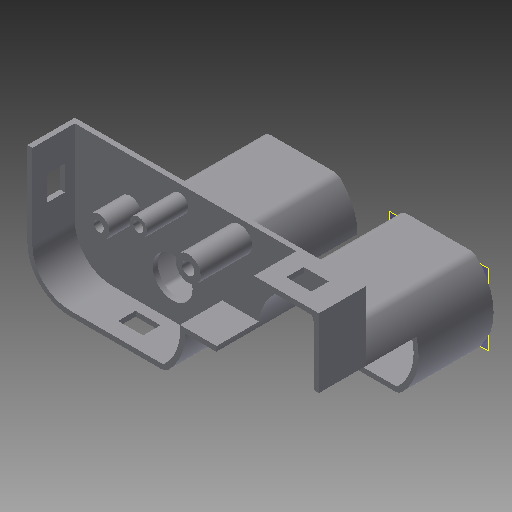
# Autodesk Inventor part: frame1
Saved by Autodesk Inventor 2017 (Build 210142000, 142)
## iProperties
Created: 2017-01-16
Part Number: frame1
Material: Generic
Document SubType Name: Modeling
Designer: Paulo Loma
Density: 1 g/cm^3
Appearance: Default
Author: Paulo Loma
Autodesk Inventor part; units mm, degrees
sketch "Sketch1" plane through (0, 0, 0) normal (0, 0, 1) x (1, 0, 0)
  arc A0 (6.9166, 7.2222) -> (6.2249, 7.5) centre (6.2249, 6.5) ccw projected
  arc A1 (6.9166, -7.2222) -> (6.9166, 7.2222) centre (0, 0) ccw
  arc A2 (6.2249, -7.5) -> (6.9166, -7.2222) centre (6.2249, -6.5) ccw projected
  line L0 (6.2249, -7.5) -> (-6.2249, -7.5)
  arc A3 (-6.9166, -7.2222) -> (-6.2249, -7.5) centre (-6.2249, -6.5) ccw projected
  arc A4 (-6.9166, 7.2222) -> (-6.9166, -7.2222) centre (0, 0) ccw
  arc A5 (-6.2249, 7.5) -> (-6.9166, 7.2222) centre (-6.2249, 6.5) ccw projected
  line L1 (-6.2249, 7.5) -> (6.2249, 7.5)
  arc A6 (-7.6083, -7.9444) -> (-6.2249, -8.5) centre (-6.2249, -6.5) ccw
  line L2 (-6.2249, -8.5) -> (6.2249, -8.5)
  arc A7 (6.2249, -8.5) -> (7.6083, -7.9444) centre (6.2249, -6.5) ccw
  arc A8 (7.6083, -7.9444) -> (7.6083, 7.9444) centre (0, 0) ccw
  arc A9 (7.6083, 7.9444) -> (6.2249, 8.5) centre (6.2249, 6.5) ccw
  line L3 (6.2249, 8.5) -> (-6.2249, 8.5)
  arc A10 (-6.2249, 8.5) -> (-7.6083, 7.9444) centre (-6.2249, 6.5) ccw
  arc A11 (-7.6083, 7.9444) -> (-7.6083, -7.9444) centre (0, 0) ccw
  dimension "d0" = 1
  constraints: 16 point on circle, 8 centre point, 8 end point, 7 other
  measures "d0" radial gap between concentric circles of A4 A11
extrude "Extrusion1" add sketch "Sketch1" against normal blind 15
sketch "Sketch2" plane through (0, 0, -15) normal (0, 0, -1) x (-1, 0, 0)
  line L0 (10.5441, 3.134) -> (9.4964, 3.1333)
  arc A0 (10.5441, 3.134) -> (7.6083, 7.9444) centre (0, 0) ccw
  arc A1 (7.6083, 7.9444) -> (6.2249, 8.5) centre (6.2249, 6.5) ccw
  line L1 (6.2249, 8.5) -> (-6.2249, 8.5)
  arc A2 (-6.2249, 8.5) -> (-7.6083, 7.9444) centre (-6.2249, 6.5) ccw
  arc A3 (-7.6083, 7.9444) -> (-11, 0) centre (0, 0) ccw
  arc A4 (9.4964, 3.1333) -> (6.9166, 7.2222) centre (0, 0) ccw
  arc A5 (6.9166, 7.2222) -> (6.2249, 7.5) centre (6.2249, 6.5) ccw
  line L2 (6.2249, 7.5) -> (-6.2249, 7.5)
  arc A6 (-6.2249, 7.5) -> (-6.9166, 7.2222) centre (-6.2249, 6.5) ccw
  arc A7 (-6.9166, 7.2222) -> (-10, 0) centre (0, 0) ccw
  arc A8 (-7.6083, 7.9444) -> (-11, 0) centre (0, 0) ccw
  line L3 (-11, 0) -> (-10, 0)
  arc A9 (-6.9166, 7.2222) -> (-10, 0) centre (0, 0) ccw
  point P0 (0, 0)
  constraints: 20 point on circle, 10 centre point, 8 end point
ref_plane "Work Plane1" through (-10.0049, -7.5065, -25) normal (0, 0, -1) x (0, 1, 0)
extrude "Extrusion2" add sketch "Sketch2" along normal up to surface (10 mm away)
sketch "Sketch3" plane through (0, 0, 0) normal (0, 0, 1) x (1, 0, 0)
  line L0 (-6.2249, -8.5) -> (6.2249, -8.5)
  arc A0 (6.2249, -8.5) -> (7.6083, -7.9444) centre (6.2249, -6.5) ccw
  arc A1 (7.6083, -7.9444) -> (11, 0) centre (0, 0) ccw
  circle A2 centre (0, 0) radius 4
  line L1 (11, 0) -> (17.2374, 0)
  line L2 (33.4623, 7.5) -> (21.0124, 7.5)
  arc A3 (21.0124, 7.5) -> (20.3208, 7.2222) centre (21.0124, 6.5) ccw
  arc A4 (20.3208, 7.2222) -> (17.2374, 0) centre (27.2374, 0) ccw
  arc A5 (34.154, 7.2222) -> (33.4623, 7.5) centre (33.4623, 6.5) ccw
  arc A6 (36.7389, 3.1179) -> (34.154, 7.2222) centre (27.2374, 0) ccw
  arc A7 (36.7389, 3.1179) -> (34.154, 7.2222) centre (27.2374, 0) ccw
  line L3 (37.7863, 3.1179) -> (36.7389, 3.1179)
  line L4 (37.7863, 3.1179) -> (37.7863, 16)
  line L5 (-20.5714, 16.9183) -> (-20.5714, 0)
  line L6 (-12.0714, -8.5) -> (6.2249, -8.5)
  line L7 (37.7863, 16.9183) -> (-20.5714, 16.9183)
  line L8 (37.7863, 16) -> (37.7863, 16.9183)
  arc A8 (-20.5714, 0) -> (-12.0714, -8.5) centre (-12.0714, 0) ccw
  point P0 (0, 0)
  point P1 (20.3297, 5.7693)
  point P2 (35.6801, 3.1179)
  constraints: 18 end point, 17 point on circle, 11 centre point, 1 tangent, 1 vertical
ref_plane "Work Plane2" through (27.2374, 0, -25) normal (0, 0, -1) x (-1, 0, 0)
sketch "Sketch4" plane through (27.2374, 0, -25) normal (0, 0, -1) x (-1, 0, 0)
  arc A0 (6.9166, 7.2222) -> (6.2249, 7.5) centre (6.2249, 6.5) ccw
  arc A1 (6.9166, -7.2222) -> (6.9166, 7.2222) centre (0, 0) ccw
  arc A2 (6.2249, -7.5) -> (6.9166, -7.2222) centre (6.2249, -6.5) ccw
  line L0 (6.2249, -7.5) -> (-6.2249, -7.5)
  arc A3 (-6.9166, -7.2222) -> (-6.2249, -7.5) centre (-6.2249, -6.5) ccw
  arc A4 (-6.9166, 7.2222) -> (-6.9166, -7.2222) centre (0, 0) ccw
  arc A5 (-6.2249, 7.5) -> (-6.9166, 7.2222) centre (-6.2249, 6.5) ccw
  line L1 (-6.2249, 7.5) -> (6.2249, 7.5)
  arc A6 (-7.6083, -7.9444) -> (-6.2249, -8.5) centre (-6.2249, -6.5) ccw
  line L2 (-6.2249, -8.5) -> (6.2249, -8.5)
  arc A7 (6.2249, -8.5) -> (7.6083, -7.9444) centre (6.2249, -6.5) ccw
  arc A8 (7.6083, -7.9444) -> (7.6083, 7.9444) centre (0, 0) ccw
  arc A9 (7.6083, 7.9444) -> (6.2249, 8.5) centre (6.2249, 6.5) ccw
  line L3 (6.2249, 8.5) -> (-6.2249, 8.5)
  arc A10 (-6.2249, 8.5) -> (-7.6083, 7.9444) centre (-6.2249, 6.5) ccw
  arc A11 (-7.6083, 7.9444) -> (-7.6083, -7.9444) centre (0, 0) ccw
  point P0 (27.2374, 0)
  dimension "d8" = 1
  constraints: 24 point on circle, 12 centre point, 8 end point, 7 other
  measures "d8" radial gap between concentric circles of A4 A11
extrude "Extrusion4" add sketch "Sketch4" against normal blind 15
sketch "Sketch5" plane through (27.2374, 0, -10) normal (0, 0, 1) x (1, 0, 0)
  line L0 (10.5489, 3.1179) -> (9.5015, 3.1179)
  line L1 (-6.2249, 7.5) -> (6.2249, 7.5)
  arc A0 (6.9166, 7.2222) -> (6.2249, 7.5) centre (6.2249, 6.5) ccw
  arc A1 (9.5015, 3.1179) -> (6.9166, 7.2222) centre (0, 0) ccw
  arc A2 (-6.9166, 7.2222) -> (-10, 0) centre (0, 0) ccw
  arc A3 (-6.2249, 7.5) -> (-6.9166, 7.2222) centre (-6.2249, 6.5) ccw
  arc A4 (10.5489, 3.1179) -> (7.6083, 7.9444) centre (0, 0) ccw
  arc A5 (7.6083, 7.9444) -> (6.2249, 8.5) centre (6.2249, 6.5) ccw
  line L2 (6.2249, 8.5) -> (-6.2249, 8.5)
  arc A6 (-6.2249, 8.5) -> (-7.6083, 7.9444) centre (-6.2249, 6.5) ccw
  arc A7 (-7.6083, 7.9444) -> (-11, 0) centre (0, 0) ccw
  arc A8 (-6.9166, 7.2222) -> (-10, 0) centre (0, 0) ccw
  line L3 (-10, 0) -> (-11, 0)
  arc A9 (-7.6083, 7.9444) -> (-11, 0) centre (0, 0) ccw
  point P0 (-27.2374, 0)
  constraints: 20 point on circle, 18 centre point, 8 end point
ref_plane "Work Plane3" through (17.2325, -7.5065, 0) normal (0, 0, 1) x (1, 0, 0)
extrude "Extrusion5" add sketch "Sketch5" along normal up to surface (10 mm away)
extrude "Extrusion6" add sketch "Sketch3" along normal blind 1
sketch "Sketch6" plane through (0, 0, 1) normal (0, 0, 1) x (1, 0, 0)
  circle A0 centre (13.4286, 13.4183) radius 2.5
  point P0 (0, 0)
  constraints: 1 centre point
ref_plane "Work Plane4" through (12.1782, 12.1679, 3.6) normal (0, 0, -1) x (0.0003267, 0.9999999, 0)
extrude "Extrusion7" add sketch "Sketch6" along normal up to surface (2.6 mm away)
sketch "Sketch7" plane through (13.4286, 13.4183, 3.6) normal (0, 0, 1) x (1, 0, 0)
  circle A0 centre (0, 0) radius 2.5 projected
  circle A1 centre (0, 0) radius 1.25 projected
  point P0 (-13.4286, -13.4183)
ref_plane "Work Plane5" through (10.1221, 10.1118, 11.3) normal (0, 0, -1) x (0.410459, 0.9118791, 0)
extrude "Extrusion8" add sketch "Sketch7" along normal up to surface (7.7 mm away)
ref_plane "Work Plane6" through (-11.501, 4.7479, 7.3) normal (0, 0, -1) x (-0.6504815, 0.7595221, 0)
ref_plane "Work Plane7" through (-1.3818, 10.8215, 9.3) normal (0, 0, -1) x (0.3848112, 0.9229953, 0)
ref_plane "Work Plane8" through (10.1221, 10.1118, 14.6) normal (0, 0, 1) x (0.9118791, -0.410459, 0)
ref_plane "Work Plane9" through (10.1221, 10.1118, 14.6) normal (0, 0, 1) x (0.9118791, -0.410459, 0)
sketch "Sketch12" plane through (0, 0, 1) normal (0, 0, 1) x (1, 0, 0)
  circle A0 centre (13.4286, 13.4183) radius 2.5
  circle A1 centre (0, 0) radius 4
  arc A2 (6.2249, -8.5) -> (7.6083, -7.9444) centre (6.2249, -6.5) ccw
  arc A3 (7.6083, -7.9444) -> (11, 0) centre (0, 0) ccw
  line L0 (11, 0) -> (17.2374, 0)
  arc A4 (20.3208, 7.2222) -> (17.2374, 0) centre (27.2374, 0) ccw
  arc A5 (21.0124, 7.5) -> (20.3208, 7.2222) centre (21.0124, 6.5) ccw
  line L1 (21.0124, 7.5) -> (33.4623, 7.5)
  arc A6 (34.154, 7.2222) -> (33.4623, 7.5) centre (33.4623, 6.5) ccw
  arc A7 (36.7389, 3.1179) -> (34.154, 7.2222) centre (27.2374, 0) ccw
  line L2 (36.7389, 3.1179) -> (37.7863, 3.1179)
  line L3 (37.7863, 3.1179) -> (37.7863, 16.9183)
  line L4 (37.7863, 16.9183) -> (-20.5714, 16.9183)
  line L5 (-20.5714, 16.9183) -> (-20.5714, 0)
  line L6 (-12.0714, -8.5) -> (6.2249, -8.5)
  line L7 (36.7389, 10.9183) -> (36.7389, 3.1179)
  line L8 (36.7389, 10.9183) -> (36.7389, 15.9183)
  line L9 (37.7863, 16.9183) -> (-20.5714, 16.9183)
  line L10 (-19.5714, 0) -> (-19.5714, 16.9183)
  line L11 (6.2249, -7.5) -> (-12.0714, -7.5)
  arc A8 (6.2249, -7.5) -> (6.9166, -7.2222) centre (6.2249, -6.5) ccw
  arc A9 (6.9166, -7.2222) -> (9.9499, 1) centre (0, 0) ccw
  line L12 (17.2875, 1) -> (9.9499, 1)
  arc A10 (-20.5714, 0) -> (-12.0714, -8.5) centre (-12.0714, 0) ccw
  arc A11 (-19.5714, 0) -> (-12.0714, -7.5) centre (-12.0714, 0) ccw
  line L13 (36.7389, 15.9183) -> (24.7389, 15.9183)
  line L14 (24.7389, 15.9183) -> (24.7389, 16.9183)
  line L15 (37.7863, 16.9183) -> (-20.5714, 16.9183) projected
  point P0 (0, 0)
  point P1 (36.7389, 16.9183)
  point P2 (-16.0714, -7.5)
  dimension "d33" = 1
  constraints: 30 end point, 23 point on circle, 19 centre point, 2 point on line, 1 perpendicular
  measures "d33" radial gap between concentric circles of A10 A11
extrude "Extrusion13" add sketch "Sketch12" along normal blind 8.5 contours L6 A10 L5 L4 L10 A11 L11 A8 A9 L12 A4 L0 A3 A2 | L4 L3 L2 L7 L8 L13 L14
sketch "Sketch13" plane through (0, 0, 1) normal (0, 0, 1) x (1, 0, 0)
  circle A0 centre (-8.4684, 7.7805) radius 2.15 projected
  point P0 (0, 0)
ref_plane "Work Plane10" through (-9.469, 6.7799, 4.9) normal (0, 0, -1) x (0, 1, 0)
extrude "Extrusion14" add sketch "Sketch13" along normal up to surface (3.9 mm away)
sketch "Sketch14" plane through (-8.4684, 7.7805, 4.9) normal (0, 0, 1) x (1, 0, 0)
  circle A0 centre (0, 0) radius 2.15 projected
  circle A1 centre (0, 0) radius 1 projected
  point P0 (8.4684, -7.7805)
ref_plane "Work Plane11" through (-11.501, 4.7479, 7.3) normal (0, 0, -1) x (-0.6504815, 0.7595221, 0)
extrude "Extrusion15" add sketch "Sketch14" along normal up to surface (2.4 mm away)
sketch "Sketch15" plane through (0, 0, 1) normal (0, 0, 1) x (1, 0, 0)
  circle A0 centre (1.4306, 13.6338) radius 1.75
  point P0 (0, 0)
  constraints: 1 centre point
ref_plane "Work Plane12" through (0.4299, 12.6331, 4.9) normal (0, 0, -1) x (0, 1, 0)
ref_plane "Work Plane13" through (-1.3818, 10.8215, 9.3) normal (0, 0, -1) x (0.3848112, 0.9229953, 0)
ref_plane "Work Plane14" through (0.4299, 12.6331, 4.9) normal (0, 0, -1) x (0, 1, 0)
extrude "Extrusion18" add sketch "Sketch15" along normal up to surface (3.9 mm away)
sketch "Sketch17" plane through (1.4306, 13.6338, 4.9) normal (0, 0, 1) x (1, 0, 0)
  circle A0 centre (0, 0) radius 1.75 projected
  circle A1 centre (0, 0) radius 1 projected
  point P0 (-1.4306, -13.6338)
ref_plane "Work Plane15" through (-1.3818, 10.8215, 9.3) normal (0, 0, -1) x (0.3848112, 0.9229953, 0)
extrude "Extrusion19" add sketch "Sketch17" along normal up to surface (4.4 mm away)
sketch "Sketch19" plane through (-6.2249, -8.5, -15) normal (0, -1, 0) x (1, 0, 0)
  line L0 (0.8017, 21.5) -> (5.8017, 21.5) projected
  line L1 (0.8017, 21.5) -> (0.8017, 18)
  line L2 (0.8017, 18) -> (5.8017, 18)
  line L3 (5.8017, 18) -> (5.8017, 21.5)
  point P0 (6.2249, 15)
  dimension "d51" = 3.5
  constraints: 6 end point, 2 perpendicular, 1 vertical
  measures "d51" distance of L0.start L1.end
extrude "Extrusion21" cut sketch "Sketch19" against normal blind 1
sketch "Sketch20" plane through (-20.5714, 0, 0) normal (-1, 0, 0) x (0, 0, 1)
  line L0 (6.5, 10.9592) -> (6.5, 5.9592) projected
  line L1 (6.5, 5.9592) -> (3, 5.9592)
  line L2 (3, 5.9592) -> (3, 10.9592)
  line L3 (3, 10.9592) -> (6.5, 10.9592)
  point P0 (0, 0)
  dimension "d54" = 3.5
  dimension "d55" = 5
  constraints: 6 end point, 1 horizontal, 1 perpendicular
  measures "d54" distance of L0.end L1.end
  measures "d55" distance of L1.end L2.end
extrude "Extrusion22" cut sketch "Sketch20" against normal blind 1
sketch "Sketch21" plane through (-20.5714, 16.9183, 0) normal (0, 1, 0) x (1, 0, 0)
  line L0 (53.8103, -6.5) -> (48.8103, -6.5) projected
  line L1 (53.8103, -6.5) -> (53.8103, -3)
  line L2 (53.8103, -3) -> (48.8103, -3)
  line L3 (48.8103, -3) -> (48.8103, -6.5)
  point P0 (20.5714, 0)
  dimension "d58" = 3.5
  constraints: 6 end point, 2 perpendicular, 1 vertical
  measures "d58" distance of L0.start L1.end
extrude "Extrusion23" cut sketch "Sketch21" against normal blind 1
body "Solid1"
